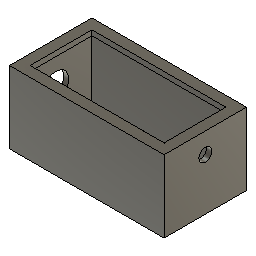
AssemblyCaseOBD (Autodesk Fusion 360 archive; units mm, degrees)
design "CaseOBDCar"
Autodesk Fusion 360 part; units mm, degrees
note: some values were not read from the file. Chosen so that the rebuilt part matches the saved one: which bodies a step acts on.
sketch "Esquisse1" plane through (0, 0, 0) normal (0, 0, 1) x (1, 0, 0)
  line L0 (0, 0) -> (150, 0)
  line L1 (150, 0) -> (150, 80)
  line L2 (150, 80) -> (0, 80)
  line L3 (0, 80) -> (0, 0)
  dimension "d1" = 150
  dimension "d2" = 80
  constraint horizontal L0
  constraint vertical L1
  constraint horizontal L2
  constraint vertical L3
  constraint coincident L0.start L3.end
  measures "d1" distance of L1.end L2.end
  measures "d2" distance of L0.end L1.end
extrude "Extrusion1" add sketch "Esquisse1" along normal blind 70
shell "Coque1" thickness 5 removed faces 0 bodies 1
sketch "Esquisse2" plane through (0, 0, 0) normal (-1, 0, 0) x (0, -1, 0)
  line L0 (-80, 0) -> (0, 0)
  line L1 (0, 0) -> (0, 70)
  line L2 (0, 70) -> (-80, 70)
  line L3 (-80, 70) -> (-80, 0)
  circle A0 centre (-40, 35) radius 12.5
  dimension "d6" = 25
  dimension "d7" = 40
  dimension "d8" = 40
  dimension "d9" = 35
  dimension "d10" = 35
  measures "d6" diameter of A0
  measures "d7" distance of L1 A0.centre
  measures "d8" distance of L3 A0.centre
  measures "d9" distance of L0 A0.centre
  measures "d10" distance of L2 A0.centre
extrude "Extrusion2" cut sketch "Esquisse2" against normal blind 20 contours A0
sketch "Esquisse3" plane through (150, 0, 0) normal (1, 0, 0) x (0, 1, 0)
  line L0 (0, 0) -> (80, 0)
  line L1 (80, 0) -> (80, 70)
  line L2 (80, 70) -> (0, 70)
  line L3 (0, 70) -> (0, 0)
  circle A0 centre (40, 50) radius 6.25
  dimension "d13" = 12.5
  dimension "d14" = 40
  dimension "d15" = 40
  dimension "d16" = 50
  measures "d13" diameter of A0
  measures "d14" distance of L1 A0.centre
  measures "d15" distance of L3 A0.centre
  measures "d16" distance of L0 A0.centre
extrude "Extrusion3" cut sketch "Esquisse3" against normal blind 15 contours A0
sketch "Esquisse4" plane through (0, 0, 70) normal (0, 0, 1) x (-1, 0, 0)
  line L0 (0, -80) -> (0, 0)
  line L1 (0, 0) -> (-150, 0)
  line L2 (-150, 0) -> (-150, -80)
  line L3 (-150, -80) -> (0, -80)
  line L4 (-10, -10) -> (-140, -10)
  line L5 (-140, -10) -> (-140, -70)
  line L6 (-140, -70) -> (-10, -70)
  line L7 (-10, -70) -> (-10, -10)
  dimension "d19" = 130
  dimension "d20" = 60
  dimension "d21" = 10
  dimension "d22" = 10
  constraint horizontal L4
  constraint vertical L5
  constraint horizontal L6
  constraint vertical L7
  measures "d19" distance of L4.start L4.end
  measures "d20" distance of L4.start L6.end
  measures "d21" distance of L0 L7
  measures "d22" distance of L1 L4
extrude "Extrusion4" cut sketch "Esquisse4" against normal blind 10 contours L4 L5 L6 L7

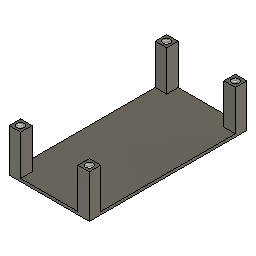
design "ESPBlock"
Autodesk Fusion 360 part; units mm, degrees
sketch "Esquisse1" plane through (0, 0, 0) normal (0, 0, 1) x (1, 0, 0)
  line L0 (0, 0) -> (28, 0)
  line L1 (28, 0) -> (28, 55)
  line L2 (28, 55) -> (0, 55)
  line L3 (0, 55) -> (0, 0)
  line L4 (28, 0) -> (24, 0)
  line L5 (24, 0) -> (24, 4)
  line L6 (24, 4) -> (28, 4)
  line L7 (28, 4) -> (28, 0)
  line L8 (0, 0) -> (4, 0)
  line L9 (4, 0) -> (4, 4)
  line L10 (4, 4) -> (0, 4)
  line L11 (0, 4) -> (0, 0)
  line L12 (0, 55) -> (4, 55)
  line L13 (4, 55) -> (4, 51)
  line L14 (4, 51) -> (0, 51)
  line L15 (0, 51) -> (0, 55)
  line L16 (28, 55) -> (24, 55)
  line L17 (24, 55) -> (24, 51)
  line L18 (24, 51) -> (28, 51)
  line L19 (28, 51) -> (28, 55)
  dimension "d1" = 55
  dimension "d2" = 28
  dimension "d3" = 4
  dimension "d4" = 4
  dimension "d5" = 4
  dimension "d6" = 4
  dimension "d7" = 4
  dimension "d8" = 4
  dimension "d9" = 4
  dimension "d10" = 4
  constraint horizontal L0
  constraint vertical L1
  constraint horizontal L2
  constraint vertical L3
  constraint coincident L0.start L3.end
  constraint horizontal L4
  constraint vertical L5
  constraint horizontal L6
  constraint vertical L7
  constraint horizontal L8
  constraint vertical L9
  constraint horizontal L10
  constraint vertical L11
  constraint horizontal L12
  constraint vertical L13
  constraint horizontal L14
  constraint vertical L15
  constraint horizontal L16
  constraint vertical L17
  constraint horizontal L18
  constraint vertical L19
  measures "d1" distance of L0.start L2.end
  measures "d2" distance of L1.end L2.end
  measures "d3" distance of L5.end L6.end
  measures "d4" distance of L4.end L5.end
  measures "d5" distance of L9.end L10.end
  measures "d6" distance of L8.end L9.end
  measures "d7" distance of L12.end L13.end
  measures "d8" distance of L13.end L14.end
  measures "d9" distance of L17.end L18.end
  measures "d10" distance of L16.end L17.end
extrude "Extrusion1" add sketch "Esquisse1" along normal blind 15 contours L0 L3 L8 L9 L10 L11 | L0 L1 L4 L5 L6 L7 | L2 L3 L12 L13 L14 L15 | L1 L2 L16 L17 L18 L19 makes body 1 at (24, 1.3333, 5) makes body 2 at (25.3333, 51, 10) makes body 3 at (0, 2.6667, 5) makes body 4 at (0, 53.6667, 5)
sketch "Esquisse2" plane through (0, 0, 0) normal (0, 0, 1) x (1, 0, 0)
  line L0 (0, 0) -> (28, 0)
  line L1 (28, 0) -> (28, 55)
  line L2 (28, 55) -> (0, 55)
  line L3 (0, 55) -> (0, 0)
  dimension "d13" = 55
  dimension "d14" = 28
  constraint horizontal L0
  constraint vertical L1
  constraint horizontal L2
  constraint vertical L3
  constraint coincident L0.start L3.end
  measures "d13" distance of L0.end L1.end
  measures "d14" distance of L0.start L0.end
extrude "Extrusion2" add sketch "Esquisse2" along normal blind 1 bodies 1 2 3 4
hole "Perçage1" at (26, 2, 15) direction (0, 0, -1) diameter 2.529 depth 8 tip angle 118 bodies 1
thread "Filetage1" "ISO Metric profile 3.0 M3x0.5 M3x0.5 6H" thread offset 0 thread depth 7.4
hole "Perçage2" at (2, 2, 15) direction (0, 0, -1) diameter 2.529 depth 8 tip angle 118 bodies 1
thread "Filetage2" "ISO Metric profile 3.0 M3x0.5 M3x0.5 6H" thread offset 0 thread depth 7.4
hole "Perçage3" at (2, 53, 15) direction (0, 0, -1) diameter 2.529 depth 8 tip angle 118 bodies 1
thread "Filetage3" "ISO Metric profile 3.0 M3x0.5 M3x0.5 6H" thread offset 0 thread depth 7.4
hole "Perçage4" at (26, 53, 15) direction (0, 0, -1) diameter 2.529 depth 8 tip angle 118 bodies 1
thread "Filetage4" "ISO Metric profile 3.0 M3x0.5 M3x0.5 6H" thread offset 0 thread depth 7.4

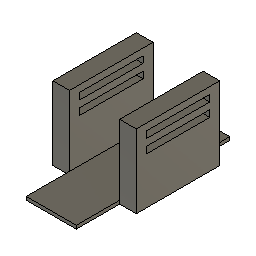
design "MAX485 Block"
Autodesk Fusion 360 part; units mm, degrees
sketch "Esquisse1" plane through (0, 0, 0) normal (0, 0, 1) x (1, 0, 0)
  line L0 (0, 0) -> (15, 0)
  line L1 (15, 0) -> (15, 46)
  line L2 (15, 46) -> (0, 46)
  line L3 (0, 46) -> (0, 0)
  dimension "d1" = 46
  dimension "d2" = 15
  constraint horizontal L0
  constraint vertical L1
  constraint horizontal L2
  constraint vertical L3
  constraint coincident L0.start L3.end
  measures "d1" distance of L0.end L1.end
  measures "d2" distance of L1.end L2.end
sketch "Esquisse2" plane through (0, 0, 0) normal (0, 0, 1) x (1, 0, 0)
  line L0 (15, 38) -> (20, 38)
  line L1 (20, 38) -> (20, 13)
  line L2 (20, 13) -> (15, 13)
  line L3 (15, 13) -> (15, 38)
  line L4 (0, 38) -> (-5, 38)
  line L5 (-5, 38) -> (-5, 13)
  line L6 (-5, 13) -> (0, 13)
  line L7 (0, 13) -> (0, 38)
  line L8 (0, 46) -> (0, 0)
  line L9 (15, 0) -> (15, 46)
  line L10 (0, 0) -> (15, 0)
  dimension "d3" = 5
  dimension "d4" = 5
  dimension "d5" = 25
  dimension "d6" = 25
  dimension "d7" = 5
  dimension "d8" = 5
  dimension "d9" = 38
  dimension "d10" = 13
  constraint horizontal L0
  constraint vertical L1
  constraint horizontal L2
  constraint vertical L3
  constraint horizontal L4
  constraint vertical L5
  constraint horizontal L6
  constraint vertical L7
  measures "d3" distance of L4.start L4.end
  measures "d4" distance of L0.start L0.end
  measures "d5" distance of L0.end L1.end
  measures "d6" distance of L4.end L5.end
  measures "d7" distance of L5 L8
  measures "d8" distance of L1 L9
  measures "d9" distance of L0 L10
  measures "d10" distance of L6 L10
extrude "Extrusion1" add sketch "Esquisse1" along normal blind 1
extrude "Extrusion2" add sketch "Esquisse2" along normal blind 22
sketch "Esquisse3" plane through (20, 0, 0) normal (1, 0, 0) x (0, 1, 0)
  line L0 (13, 0) -> (38, 0)
  line L1 (38, 0) -> (38, 22)
  line L2 (38, 22) -> (13, 22)
  line L3 (13, 22) -> (13, 0)
  line L4 (16, 20) -> (35, 20)
  line L5 (35, 20) -> (35, 18)
  line L6 (35, 18) -> (16, 18)
  line L7 (16, 18) -> (16, 20)
  line L8 (16, 16) -> (35, 16)
  line L9 (35, 16) -> (35, 14)
  line L10 (35, 14) -> (16, 14)
  line L11 (16, 14) -> (16, 16)
  dimension "d15" = 3
  dimension "d16" = 3
  dimension "d17" = 19
  dimension "d18" = 2
  dimension "d19" = 2
  dimension "d20" = 2
  dimension "d21" = 19
  dimension "d22" = 3
  dimension "d23" = 2
  constraint horizontal L4
  constraint vertical L5
  constraint horizontal L6
  constraint vertical L7
  constraint horizontal L8
  constraint vertical L9
  constraint horizontal L10
  constraint vertical L11
  measures "d15" distance of L3 L7
  measures "d16" distance of L1 L5
  measures "d17" distance of L5.end L6.end
  measures "d18" distance of L4.end L5.end
  measures "d19" distance of L2 L4
  measures "d20" distance of L8.end L9.end
  measures "d21" distance of L9.end L10.end
  measures "d22" distance of L1 L9
  measures "d23" distance of L6 L8
extrude "Extrusion3" cut sketch "Esquisse3" against normal blind 25 contours L4 L5 L6 L7 | L8 L9 L10 L11
